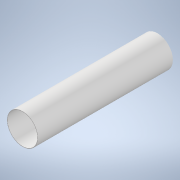
# Autodesk Inventor part: 4.5 inch diameter pipe
Saved by Autodesk Inventor 2021 (Build 250183000, 183)
## iProperties
Created: 2022-05-23
Part Number: 4.5 inch diameter pipe
Material: Generic
Document SubType Name: Modeling
Designer: techv
Density: 1 g/cm^3
Appearance: Default
Author: techv
Autodesk Inventor part; units mm, degrees
ref_plane "YZ Plane" through (0, 0, 0) normal (1, 0, 0) x (0, 1, 0)
ref_plane "XZ Plane" through (0, 0, 0) normal (0, 1, 0) x (-1, 0, 0)
ref_plane "XY Plane" through (0, 0, 0) normal (0, 0, 1) x (1, 0, 0)
sketch "Sketch1" plane through (0, 0, 0) normal (0, 0, 1) x (1, 0, 0)
  circle A0 centre (0, -59.15) radius 57.15 projected
  circle A1 centre (0, -59.15) radius 59.15 projected
  circle A2 centre (0, -59.15) radius 55.15
  point P0 (0, 0)
  dimension "d0" = 110.3
  constraints: 1 centre point, 1 coincident, 1 vertical alignment
  measures "d0" diameter of A2
extrude "Extrusion1" add sketch "Sketch1" along normal blind 500 contours A0
body "Solid1"
